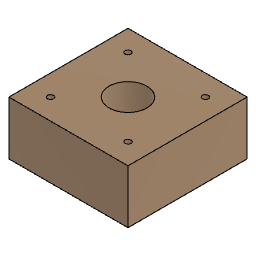
X platform support base (Autodesk Fusion 360 design; units mm, degrees)
Autodesk Fusion 360 part; units mm, degrees
sketch "Base" plane through (0, 0, 0) normal (0, 0, 1) x (1, 0, 0)
  line L0 (20, 20) -> (-20, 20)
  line L1 (-20, 20) -> (-20, -20)
  line L2 (-20, -20) -> (20, -20)
  line L3 (20, -20) -> (20, 20)
  line L4 (20, 20) -> (-20, -20) construction
  line L5 (-20, 20) -> (20, -20) construction
  circle A0 centre (0, 0) radius 2
  circle A1 centre (0, 0) radius 6.35
  line L6 (13, 13) -> (-13, 13) construction
  line L7 (-13, 13) -> (-13, -13) construction
  line L8 (-13, -13) -> (13, -13) construction
  line L9 (13, -13) -> (13, 13) construction
  line L10 (13, 13) -> (-13, -13) construction
  line L11 (-13, 13) -> (13, -13) construction
  circle A2 centre (-13, 13) radius 1
  circle A3 centre (13, 13) radius 1
  circle A4 centre (13, -13) radius 1
  circle A5 centre (-13, -13) radius 1
  dimension "d1" = 40
  dimension "d2" = 40
  dimension "d3" = 4
  dimension "d6" = 12.7
  dimension "d10" = 26
  dimension "d11" = 26
  dimension "d12" = 2
  dimension "d13" = 2
  dimension "d14" = 2
  dimension "d15" = 2
  constraint perpendicular L0 L1
  constraint parallel L0 L2
  constraint parallel L1 L3
  constraint horizontal L0
  constraint coincident L4 A0.centre
  constraint coincident L5 A0.centre
  constraint coincident A0.centre A1.centre
  constraint perpendicular L6 L7
  constraint parallel L6 L8
  constraint parallel L7 L9
  constraint horizontal L6
  constraint coincident L10 A0.centre
  constraint coincident L11 A0.centre
  constraint coincident L6.end L7.start
  constraint coincident L6.start L9.end
  constraint coincident L8.end L9.start
  constraint coincident L7.end L8.start
  measures "d1" distance of L1.end L2.end
  measures "d2" distance of L0.end L1.end
  measures "d3" diameter of A0
  measures "d6" diameter of A1
  measures "d10" distance of L7.end L8.end
  measures "d11" distance of L6.end L7.end
  measures "d12" diameter of A2
  measures "d13" diameter of A3
  measures "d14" diameter of A4
  measures "d15" diameter of A5
extrude "Extrude1" add sketch "Base" along normal blind 18 contours L0 L1 L2 L3
extrude "Extrude2" add sketch "Base" along normal blind 9 contours A1
chamfer "Chamfer1" distance 2.5 angle 45 1 edges at (-1.8647, 0.7232, 9)
equation "d13 = d12"
equation "d14 = d12"
equation "d15 = d12"
named bodies: "Support base"
